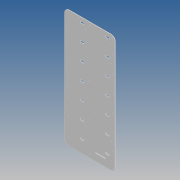
# Autodesk Inventor part: back_Box
Saved by Autodesk Inventor 2020 (Build 240168000, 168)
## iProperties
Created: 2020-07-14
Part Number: back_Box
Material: Générique
Document SubType Name: Modeling
Designer: carmine.arcudi
Density: 1 g/cm^3
Appearance: Par défaut
Author: carmine.arcudi
Autodesk Inventor part; units mm, degrees
ref_plane "YZ Plane" through (0, 0, 0) normal (1, 0, 0) x (0, 1, 0)
ref_plane "XZ Plane" through (0, 0, 0) normal (0, 1, 0) x (-1, 0, 0)
ref_plane "XY Plane" through (0, 0, 0) normal (0, 0, 1) x (1, 0, 0)
sketch "Esquisse1" plane through (0, 0, 0) normal (0, 0, 1) x (1, 0, 0)
  line L0 (-120, 336) -> (120, 336)
  line L1 (144, 312) -> (144, -312)
  line L2 (120, -336) -> (-120, -336)
  line L3 (-144, -312) -> (-144, 312)
  circle A0 centre (121, -288) radius 1.25
  circle A1 centre (24, -288) radius 1.25
  line L4 (90.6, -260) -> (110.6, -260)
  line L5 (110.6, -260) -> (110.6, -270)
  line L6 (110.6, -270) -> (90.6, -270)
  line L7 (90.6, -270) -> (90.6, -260)
  line L8 (90.6, -164) -> (110.6, -164)
  line L9 (110.6, -164) -> (110.6, -174)
  line L10 (90.6, -174) -> (90.6, -164)
  line L11 (110.6, -174) -> (90.6, -174)
  circle A2 centre (24, -192) radius 1.25
  circle A3 centre (121, -192) radius 1.25
  line L12 (90.6, -68) -> (110.6, -68)
  line L13 (110.6, -68) -> (110.6, -78)
  line L14 (90.6, -78) -> (90.6, -68)
  line L15 (110.6, -78) -> (90.6, -78)
  circle A4 centre (24, -96) radius 1.25
  circle A5 centre (121, -96) radius 1.25
  line L16 (90.6, 28) -> (110.6, 28)
  line L17 (110.6, 28) -> (110.6, 18)
  line L18 (90.6, 18) -> (90.6, 28)
  line L19 (110.6, 18) -> (90.6, 18)
  circle A6 centre (24, 0) radius 1.25
  circle A7 centre (121, 0) radius 1.25
  line L20 (90.6, 124) -> (110.6, 124)
  line L21 (110.6, 124) -> (110.6, 114)
  line L22 (90.6, 114) -> (90.6, 124)
  line L23 (110.6, 114) -> (90.6, 114)
  circle A8 centre (24, 96) radius 1.25
  circle A9 centre (121, 96) radius 1.25
  line L24 (90.6, 220) -> (110.6, 220)
  line L25 (110.6, 220) -> (110.6, 210)
  line L26 (90.6, 210) -> (90.6, 220)
  line L27 (110.6, 210) -> (90.6, 210)
  circle A10 centre (24, 192) radius 1.25
  circle A11 centre (121, 192) radius 1.25
  line L28 (90.6, 316) -> (110.6, 316)
  line L29 (110.6, 316) -> (110.6, 306)
  line L30 (90.6, 306) -> (90.6, 316)
  line L31 (110.6, 306) -> (90.6, 306)
  circle A12 centre (24, 288) radius 1.25
  circle A13 centre (121, 288) radius 1.25
  line L32 (-53.4, -260) -> (-33.4, -260)
  line L33 (-33.4, -260) -> (-33.4, -270)
  line L34 (-53.4, -270) -> (-53.4, -260)
  line L35 (-33.4, -270) -> (-53.4, -270)
  circle A14 centre (-120, -288) radius 1.25
  circle A15 centre (-23, -288) radius 1.25
  line L36 (-53.4, -164) -> (-33.4, -164)
  line L37 (-33.4, -164) -> (-33.4, -174)
  line L38 (-53.4, -174) -> (-53.4, -164)
  line L39 (-33.4, -174) -> (-53.4, -174)
  circle A16 centre (-120, -192) radius 1.25
  circle A17 centre (-23, -192) radius 1.25
  line L40 (-53.4, -68) -> (-33.4, -68)
  line L41 (-33.4, -68) -> (-33.4, -78)
  line L42 (-53.4, -78) -> (-53.4, -68)
  line L43 (-33.4, -78) -> (-53.4, -78)
  circle A18 centre (-120, -96) radius 1.25
  circle A19 centre (-23, -96) radius 1.25
  line L44 (-53.4, 28) -> (-33.4, 28)
  line L45 (-33.4, 28) -> (-33.4, 18)
  line L46 (-53.4, 18) -> (-53.4, 28)
  line L47 (-33.4, 18) -> (-53.4, 18)
  circle A20 centre (-120, 0) radius 1.25
  circle A21 centre (-23, 0) radius 1.25
  line L48 (-53.4, 124) -> (-33.4, 124)
  line L49 (-33.4, 124) -> (-33.4, 114)
  line L50 (-53.4, 114) -> (-53.4, 124)
  line L51 (-33.4, 114) -> (-53.4, 114)
  circle A22 centre (-120, 96) radius 1.25
  circle A23 centre (-23, 96) radius 1.25
  line L52 (-53.4, 220) -> (-33.4, 220)
  line L53 (-33.4, 220) -> (-33.4, 210)
  line L54 (-53.4, 210) -> (-53.4, 220)
  line L55 (-33.4, 210) -> (-53.4, 210)
  circle A24 centre (-120, 192) radius 1.25
  circle A25 centre (-23, 192) radius 1.25
  line L56 (-53.4, 316) -> (-33.4, 316)
  line L57 (-33.4, 316) -> (-33.4, 306)
  line L58 (-53.4, 306) -> (-53.4, 316)
  line L59 (-33.4, 306) -> (-53.4, 306)
  circle A26 centre (-120, 288) radius 1.25
  circle A27 centre (-23, 288) radius 1.25
  circle A28 centre (130, -322) radius 1.25
  circle A29 centre (130, 322) radius 1.25
  circle A30 centre (0, -322) radius 1.25
  circle A31 centre (0, 322) radius 1.25
  circle A32 centre (-130, -322) radius 1.25
  circle A33 centre (-130, 322) radius 1.25
  circle A34 centre (130, -240) radius 1.25
  circle A35 centre (130, -144) radius 1.25
  circle A36 centre (130, -48) radius 1.25
  circle A37 centre (130, 48) radius 1.25
  circle A38 centre (130, 144) radius 1.25
  circle A39 centre (130, 240) radius 1.25
  circle A40 centre (0, -240) radius 1.25
  circle A41 centre (0, -144) radius 1.25
  circle A42 centre (0, -48) radius 1.25
  circle A43 centre (0, 48) radius 1.25
  circle A44 centre (0, 144) radius 1.25
  circle A45 centre (0, 240) radius 1.25
  circle A46 centre (-130, -240) radius 1.25
  circle A47 centre (-130, -144) radius 1.25
  circle A48 centre (-130, -48) radius 1.25
  circle A49 centre (-130, 48) radius 1.25
  circle A50 centre (-130, 144) radius 1.25
  circle A51 centre (-130, 240) radius 1.25
  arc A52 (-120, 336) -> (-144, 312) centre (-120, 312) ccw
  arc A53 (144, 312) -> (120, 336) centre (120, 312) ccw
  arc A54 (-144, -312) -> (-120, -336) centre (-120, -312) ccw
  arc A55 (120, -336) -> (144, -312) centre (120, -312) ccw
  line L60 (34, -290) -> (88, -290)
  line L61 (88, -290) -> (88, -296)
  line L62 (88, -296) -> (34, -296)
  line L63 (34, -296) -> (34, -290)
  circle A56 centre (32, -293) radius 1.375
  circle A57 centre (90, -293) radius 1.375
  point P0 (0, 0)
  point P1 (-144, 336)
  point P2 (144, 336)
  point P3 (-144, -336)
  dimension "d0" = 288
  dimension "d1" = 672
  dimension "d2" = 144
  dimension "d3" = 336
  dimension "d4" = 2.5
  dimension "d5" = 2.5
  dimension "d6" = 97
  dimension "d7" = 48
  dimension "d8" = 48
  dimension "d9" = 23
  dimension "d10" = 20
  dimension "d11" = 10
  dimension "d12" = 33.4
  dimension "d13" = 66
  dimension "d16" = 96
  dimension "d19" = 144
  dimension "d22" = 2.5
  dimension "d23" = 14
  dimension "d24" = 14
  dimension "d27" = 644
  dimension "d30" = 130
  dimension "d33" = 2.5
  dimension "d34" = 14
  dimension "d35" = 96
  dimension "d38" = 96
  dimension "d41" = 130
  dimension "d44" = 24
  dimension "d45" = 24
  dimension "d46" = 24
  dimension "d47" = 24
  dimension "d48" = 54
  dimension "d49" = 6
  dimension "d50" = 2.75
  dimension "d51" = 2.75
  dimension "d52" = 3
  dimension "d53" = 3
  dimension "d54" = 58
  dimension "d55" = 2
  dimension "d56" = 40
  dimension "d57" = 56
  constraints: 128 end point, 58 centre point, 8 point on circle, 8 tangent, 6 horizontal, 6 parallel, 6 point on line, 3 perpendicular, 3 vertical, 200 other
  measures "d0" distance of point (-144, 336) point (144, 336)
  measures "d1" distance of point (-144, -336) point (-144, 336)
  measures "d2" distance from line of L3 point (0, 0)
  measures "d3" distance from line of point (0, 0) L0
  measures "d4" diameter of A0
  measures "d5" diameter of A1
  measures "d6" distance of A0.centre A1.centre
  measures "d7" distance from line of A1.centre L2
  measures "d8" distance from line of A0.centre L2
  measures "d9" distance from line of L1 A0.centre
  measures "d10" distance of L4.start L4.end
  measures "d11" distance of L6.end L4.start
  measures "d12" distance between parallel lines of L1 L5
  measures "d13" distance between parallel lines of L6 L2
  measures "d16" distance of L4.start L8.start
  measures "d19" distance of L4.start L32.start
  measures "d22" diameter of A28
  measures "d23" distance from line of A28.centre L2
  measures "d24" distance from line of L1 A28.centre
  measures "d27" distance of A28.centre A29.centre
  measures "d30" distance of A28.centre A30.centre
  measures "d33" diameter of A34
  measures "d34" distance from line of L1 A34.centre
  measures "d35" distance from line of L2 A34.centre
  measures "d38" distance of A34.centre A35.centre
  measures "d41" distance of A34.centre A40.centre
  measures "d44" radius of A52
  measures "d45" radius of A53
  measures "d46" radius of A54
  measures "d47" radius of A55
  measures "d48" distance of L60.start L60.end
  measures "d49" distance of L60.end L61.end
  measures "d50" diameter of A56
  measures "d51" diameter of A57
  measures "d52" distance from line of L62 A56.centre
  measures "d53" distance from line of A57.centre L62
  measures "d54" distance of A57.centre A56.centre
  measures "d55" distance from line of L63 A56.centre
  measures "d56" distance between parallel lines of L62 L2
  measures "d57" distance between parallel lines of L1 L61
extrude "Extrusion1" add sketch "Esquisse1" along normal blind 3
equation "\"d2\" = 0.5 * d0"
equation "\"d3\" = 0.5 * d1"
equation "\"d51\" = d50"
equation "\"d52\" = 0.5 * d49"
equation "\"d53\" = 0.5 * d49"
equation "\"d55\" = -0.5 * d48 + 0.5 * d54"
